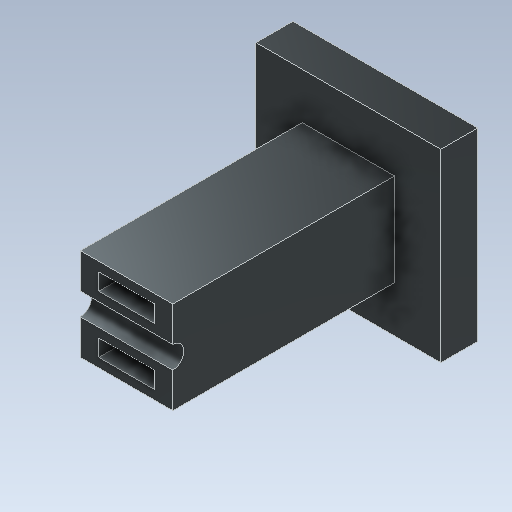
# Autodesk Inventor part: laser bottom
Saved by Autodesk Inventor 2021 (Build 250183000, 183)
## iProperties
Created: 2021-06-12
Part Number: laser bottom
Material: Iron, Cast
Document SubType Name: Modeling
Designer: user
Density: 7.15 g/cm^3
Appearance: Iron Gray
Author: user
Autodesk Inventor part; units mm, degrees
ref_plane "YZ Plane" through (0, 0, 0) normal (1, 0, 0) x (0, 1, 0)
ref_plane "XZ Plane" through (0, 0, 0) normal (0, 1, 0) x (-1, 0, 0)
ref_plane "XY Plane" through (0, 0, 0) normal (0, 0, 1) x (1, 0, 0)
sketch "Sketch1" plane through (0, 0, 0) normal (0, 0, 1) x (1, 0, 0)
  line L0 (-45.4918, 50) -> (54.5082, 50)
  line L1 (54.5082, 50) -> (54.5082, -50)
  line L2 (54.5082, -50) -> (-45.4918, -50)
  line L3 (-45.4918, -50) -> (-45.4918, 50)
  point P0 (0, 0)
  dimension "d0" = 100
  dimension "d1" = 100
  constraints: 8 end point, 2 parallel, 1 horizontal, 1 perpendicular
  measures "d0" distance of L0.start L0.end
  measures "d1" distance of L2.end L0.start
extrude "Extrusion1" add sketch "Sketch1" along normal blind 20
sketch "Sketch2" plane through (0, 0, 20) normal (0, 0, 1) x (1, 0, 0)
  line L0 (-20.4918, 25) -> (29.5082, 25)
  line L1 (29.5082, 25) -> (29.5082, -25)
  line L2 (29.5082, -25) -> (-20.4918, -25)
  line L3 (-20.4918, -25) -> (-20.4918, 25)
  line L4 (54.5082, 50) -> (-45.4918, 50) projected
  line L5 (-45.4918, 50) -> (-45.4918, -50) projected
  line L6 (-45.4918, -50) -> (54.5082, -50) projected
  line L7 (54.5082, -50) -> (54.5082, 50) projected
  point P0 (0, 0)
  dimension "d4" = 25
  dimension "d5" = 25
  dimension "d6" = 25
  dimension "d7" = 25
  constraints: 8 end point, 2 parallel, 1 horizontal, 1 perpendicular
  measures "d4" distance between parallel lines of L4 L0
  measures "d5" distance between parallel lines of L5 L3
  measures "d6" distance between parallel lines of L6 L2
  measures "d7" distance between parallel lines of L7 L1
extrude "Extrusion2" add sketch "Sketch2" along normal blind 120 contours L0 L1 L2 L3
sketch "Sketch3" plane through (29.5082, -25, 20) normal (1, 0, 0) x (0, 0, -1)
  line L0 (-120, 50) -> (-120, 0) projected
  circle A0 centre (-120, 25) radius 6
  point P0 (20, 25)
  dimension "d10" = 12
  constraints: 1 centre point, 1 midpoint
  measures "d10" diameter of A0
extrude "Extrusion3" cut sketch "Sketch3" against normal blind 50
sketch "Sketch4" plane through (0, 0, 140) normal (0, 0, 1) x (1, 0, 0)
  line L0 (19.5082, -11) -> (-10.4918, -11)
  line L1 (-10.4918, -11) -> (-10.4918, -20)
  line L2 (-10.4918, -20) -> (19.5082, -20)
  line L3 (19.5082, -20) -> (19.5082, -11)
  line L4 (19.5082, 20) -> (-10.4918, 20)
  line L5 (-10.4918, 20) -> (-10.4918, 11)
  line L6 (-10.4918, 11) -> (19.5082, 11)
  line L7 (19.5082, 11) -> (19.5082, 20)
  line L8 (29.5082, 6) -> (29.5082, 25) projected
  line L9 (-20.4918, 25) -> (-20.4918, 6) projected
  line L10 (29.5082, 25) -> (-20.4918, 25) projected
  line L11 (-20.4918, 6) -> (29.5082, 6) projected
  line L12 (29.5082, -6) -> (-20.4918, -6) projected
  line L13 (-20.4918, -25) -> (29.5082, -25) projected
  point P0 (0, 0)
  dimension "d13" = 10
  dimension "d14" = 10
  dimension "d15" = 5
  dimension "d16" = 5
  dimension "d17" = 5
  dimension "d18" = 5
  constraints: 16 end point, 4 parallel, 2 horizontal, 2 perpendicular, 2 point on line
  measures "d13" distance between parallel lines of L8 L7
  measures "d14" distance between parallel lines of L9 L5
  measures "d15" distance between parallel lines of L10 L4
  measures "d16" distance between parallel lines of L11 L6
  measures "d17" distance between parallel lines of L12 L0
  measures "d18" distance between parallel lines of L13 L2
extrude "Extrusion4" cut sketch "Sketch4" against normal blind 20 contours L3 L2 L1 L0 | L7 L6 L5 L4
equation "\"d1\" = d0"
equation "\"d5\" = d4"
equation "\"d6\" = d4"
equation "\"d7\" = d4"
body "Solid1"
